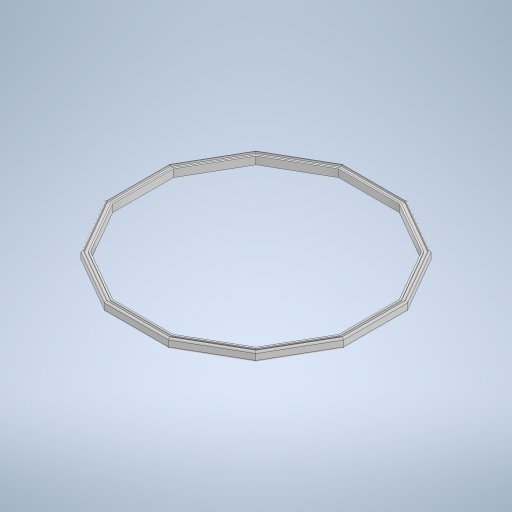
# Autodesk Inventor part: (x2)_POSPA_Large_Bottom
Saved by Autodesk Inventor 2024 (Build 280153000, 153)
## iProperties
Created: 2023-12-08
Part Number: (x2)_POSPA_Large_Bottom
Material: 일반
Document SubType Name: Modeling
Designer: jsw
Density: 1 g/cm^3
Appearance: 기본값
Author: jsw
Autodesk Inventor part; units mm, degrees
ref_plane "YZ Plane" through (0, 0, 0) normal (1, 0, 0) x (0, 1, 0)
ref_plane "XZ Plane" through (0, 0, 0) normal (0, 1, 0) x (-1, 0, 0)
sketch "스케치1" plane through (0, 0, 0) normal (0, 1, 0) x (-1, 0, 0)
  line L0 (-62.3615, 62.3615) -> (-22.8259, 85.1874)
  line L1 (-22.8259, 85.1874) -> (22.8259, 85.1874)
  line L2 (22.8259, 85.1874) -> (62.3615, 62.3615)
  line L3 (62.3615, 62.3615) -> (85.1874, 22.8259)
  line L4 (85.1874, 22.8259) -> (85.1874, -22.8259)
  line L5 (85.1874, -22.8259) -> (62.3615, -62.3615)
  line L6 (62.3615, -62.3615) -> (22.8259, -85.1874)
  line L7 (22.8259, -85.1874) -> (-22.8259, -85.1874)
  line L8 (-22.8259, -85.1874) -> (-62.3615, -62.3615)
  line L9 (-62.3615, -62.3615) -> (-85.1874, -22.8259)
  line L10 (-85.1874, -22.8259) -> (-85.1874, 22.8259)
  line L11 (-85.1874, 22.8259) -> (-62.3615, 62.3615)
  line L12 (88.3874, -23.6833) -> (64.7041, -64.7041)
  line L13 (64.7041, -64.7041) -> (23.6833, -88.3874)
  line L14 (23.6833, -88.3874) -> (-23.6833, -88.3874)
  line L15 (-23.6833, -88.3874) -> (-64.7041, -64.7041)
  line L16 (-64.7041, -64.7041) -> (-88.3874, -23.6833)
  line L17 (-88.3874, -23.6833) -> (-88.3874, 23.6833)
  line L18 (-88.3874, 23.6833) -> (-64.7041, 64.7041)
  line L19 (-64.7041, 64.7041) -> (-23.6833, 88.3874)
  line L20 (-23.6833, 88.3874) -> (23.6833, 88.3874)
  line L21 (23.6833, 88.3874) -> (64.7041, 64.7041)
  line L22 (64.7041, 64.7041) -> (88.3874, 23.6833)
  line L23 (88.3874, 23.6833) -> (88.3874, -23.6833)
  point P0 (0, 0)
  point P1 (0, 0)
  point P2 (0, 0)
  dimension "d0" = 176.385
  dimension "d1" = 3.2
  constraints: 48 end point, 2 coincident, 2 horizontal, 50 other
  measures "d0" distance of L8.end L2.end
  measures "d1" distance between parallel lines of L3 L22
extrude "돌출1" add sketch "스케치1" along normal blind 6.8 contours L0 L1 L2 L3 L4 L5 L6 L7 L8 L9 L10 L11 | L12 L13 L14 L15 L16 L17 L18 L19 L20 L21 L22 L23
sketch "스케치2" plane through (0, 6.8, 0) normal (0, 1, 0) x (1, 0, 0)
  line L0 (-23.2546, 86.7874) -> (23.2546, 86.7874)
  line L1 (23.2546, 86.7874) -> (63.5328, 63.5328)
  line L2 (63.5328, 63.5328) -> (86.7874, 23.2546)
  line L3 (86.7874, 23.2546) -> (86.7874, -23.2546)
  line L4 (86.7874, -23.2546) -> (63.5328, -63.5328)
  line L5 (63.5328, -63.5328) -> (23.2546, -86.7874)
  line L6 (23.2546, -86.7874) -> (-23.2546, -86.7874)
  line L7 (-23.2546, -86.7874) -> (-63.5328, -63.5328)
  line L8 (-63.5328, -63.5328) -> (-86.7874, -23.2546)
  line L9 (-86.7874, -23.2546) -> (-86.7874, 23.2546)
  line L10 (-86.7874, 23.2546) -> (-63.5328, 63.5328)
  line L11 (-63.5328, 63.5328) -> (-23.2546, 86.7874)
  line L12 (-88.3874, 23.6833) -> (-88.3874, -23.6833) projected
  line L13 (22.7187, -84.7874) -> (-22.7187, -84.7874)
  line L14 (-22.7187, -84.7874) -> (-62.0687, -62.0687)
  line L15 (-62.0687, -62.0687) -> (-84.7874, -22.7187)
  line L16 (-84.7874, -22.7187) -> (-84.7874, 22.7187)
  line L17 (-84.7874, 22.7187) -> (-62.0687, 62.0687)
  line L18 (-62.0687, 62.0687) -> (-22.7187, 84.7874)
  line L19 (-22.7187, 84.7874) -> (22.7187, 84.7874)
  line L20 (22.7187, 84.7874) -> (62.0687, 62.0687)
  line L21 (62.0687, 62.0687) -> (84.7874, 22.7187)
  line L22 (84.7874, 22.7187) -> (84.7874, -22.7187)
  line L23 (84.7874, -22.7187) -> (62.0687, -62.0687)
  line L24 (62.0687, -62.0687) -> (22.7187, -84.7874)
  point P0 (0, 0)
  point P1 (0, 0)
  point P2 (0, 0)
  dimension "d4" = 1.6
  dimension "d5" = 2
  constraints: 48 end point, 2 coincident, 2 horizontal, 50 other
  measures "d4" distance between parallel lines of L9 L12
  measures "d5" distance between parallel lines of L16 L9
extrude "돌출2" cut sketch "스케치2" against normal blind 1.2
sketch "스케치5" plane through (0, 6.8, 0) normal (0, 1, 0) x (1, 0, 0)
  line L0 (-62.0687, -62.0687) -> (-22.7187, -84.7874) projected
  line L1 (-22.7187, -84.7874) -> (22.7187, -84.7874) projected
  line L2 (22.7187, -84.7874) -> (62.0687, -62.0687) projected
  line L3 (62.0687, -62.0687) -> (84.7874, -22.7187) projected
  line L4 (84.7874, -22.7187) -> (84.7874, 22.7187) projected
  line L5 (84.7874, 22.7187) -> (62.0687, 62.0687) projected
  line L6 (62.0687, 62.0687) -> (22.7187, 84.7874) projected
  line L7 (22.7187, 84.7874) -> (-22.7187, 84.7874) projected
  line L8 (-22.7187, 84.7874) -> (-62.0687, 62.0687) projected
  line L9 (-62.0687, 62.0687) -> (-84.7874, 22.7187) projected
  line L10 (-84.7874, 22.7187) -> (-84.7874, -22.7187) projected
  line L11 (-84.7874, -22.7187) -> (-62.0687, -62.0687) projected
  point P0 (0, 0)
extrude "돌출5" cut sketch "스케치5" against normal blind 0.6
fillet "모깎기1" radius 1.2 24 edges at (76.5457, 0, 44.1937) (76.5457, 6.8, 44.1937) (88.3874, 6.8, 0) (88.3874, 0, 0) (76.5457, 6.8, -44.1937) (76.5457, 0, -44.1937) (44.1937, 6.8, -76.5457) (44.1937, 0, -76.5457) (0, 0, -88.3874) (0, 6.8, -88.3874) (-44.1937, 6.8, -76.5457) (-44.1937, 0, -76.5457) (-76.5457, 0, -44.1937) (-76.5457, 6.8, -44.1937) (-88.3874, 0, 0) (-88.3874, 6.8, 0) (-76.5457, 0, 44.1937) (-76.5457, 6.8, 44.1937) (-44.1937, 0, 76.5457) (-44.1937, 6.8, 76.5457) (0, 0, 88.3874) (0, 6.8, 88.3874) (44.1937, 0, 76.5457) (44.1937, 6.8, 76.5457)
ref_plane "작업 평면1" through (0, 3.4, 0) normal (0, -1, 0) x (1, 0, 0)
mirror "미러1" about plane through (0, 3.4, 0) normal (0, -1, 0) of "돌출5", "돌출2"
sketch "스케치9" plane through (-22.7187, 0.6, 84.7874) normal (0, -1, 0) x (1, 0, 0)
  line L0 (0.3215, -168.3748) -> (-38.4715, -145.9776)
  line L1 (-38.4715, -145.9776) -> (-60.8687, -107.1846)
  line L2 (-60.8687, -107.1846) -> (-60.8687, -62.3902)
  line L3 (-60.8687, -62.3902) -> (-38.4715, -23.5972)
  line L4 (-38.4715, -23.5972) -> (0.3215, -1.2)
  line L5 (0.3215, -1.2) -> (45.1159, -1.2)
  line L6 (45.1159, -1.2) -> (83.909, -23.5972)
  line L7 (83.909, -23.5972) -> (106.3061, -62.3902)
  line L8 (106.3061, -62.3902) -> (106.3061, -107.1846)
  line L9 (106.3061, -107.1846) -> (83.909, -145.9776)
  line L10 (83.909, -145.9776) -> (45.1159, -168.3748)
  line L11 (45.1159, -168.3748) -> (0.3215, -168.3748)
  line L12 (107.5061, -62.0687) -> (107.5061, -107.5061) projected
  point P0 (22.7187, -84.7874)
  point P1 (22.7187, -84.7874)
  dimension "d37" = 1.2
  constraints: 24 end point, 1 coincident, 1 horizontal, 25 other
  measures "d37" distance between parallel lines of L8 L12
extrude "돌출9" cut sketch "스케치9" against normal blind 10
